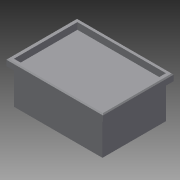
# Autodesk Inventor part: LED_BUTTON
Saved by Autodesk Inventor 2015 (Build 190159000, 159)
## iProperties
Created: 2015-02-07
Part Number: LED_BUTTON
Material: Generic
Document SubType Name: Modeling
Designer: lucanao16
Density: 1 g/cm^3
Appearance: Default
Author: lucanao16
Autodesk Inventor part; units mm, degrees
ref_plane "YZ Plane" through (0, 0, 0) normal (1, 0, 0) x (0, 1, 0)
ref_plane "XZ Plane" through (0, 0, 0) normal (0, 1, 0) x (-1, 0, 0)
ref_plane "XY Plane" through (0, 0, 0) normal (0, 0, 1) x (1, 0, 0)
sketch "Sketch1" plane through (0, 0, 0) normal (0, 1, 0) x (-1, 0, 0)
  line L0 (0, 0) -> (21.9964, 0)
  line L1 (21.9964, 0) -> (21.9964, -15.7734)
  line L2 (21.9964, -15.7734) -> (0, -15.7734)
  line L3 (0, -15.7734) -> (0, 0)
  dimension "d0" = 21.9964
  dimension "d1" = 15.7734
  constraints: 8 end point, 2 parallel, 1 horizontal, 1 perpendicular
  measures "d0" distance of L1.end L2.end
  measures "d1" distance of L0.end L1.end
extrude "Extrusion1" add sketch "Sketch1" along normal blind 8.6868
sketch "Sketch2" plane through (0, 8.6868, 0) normal (0, 1, 0) x (1, 0, 0)
  line L0 (-21.9964, 0) -> (0, 0) projected
  line L1 (0, 0) -> (0, 15.7734) projected
  line L2 (0, 15.7734) -> (-21.9964, 15.7734) projected
  line L3 (-21.9964, 15.7734) -> (-21.9964, 0) projected
  line L4 (-10.9982, 7.8867) -> (-10.9982, 16.6751)
  line L5 (-10.9982, 7.8867) -> (-22.9997, 7.8867)
  line L6 (-22.9997, 16.6751) -> (1.0287, 16.6751)
  line L7 (1.0287, 16.6751) -> (1.0287, -0.9017)
  line L8 (1.0287, -0.9017) -> (-22.9997, -0.9017)
  line L9 (-22.9997, -0.9017) -> (-22.9997, 16.6751)
  dimension "d4" = 8.7884
  dimension "d5" = 12.0015
  dimension "d6" = 24.0284
  dimension "d7" = 17.5768
  dimension "d8" = 0
  dimension "d9" = 7.8867
  constraints: 12 end point, 2 horizontal, 2 parallel, 1 perpendicular, 1 vertical
  measures "d4" distance of L4.start L4.end
  measures "d5" distance of L4.start L5.end
  measures "d6" distance of L7.end L8.end
  measures "d7" distance of L6.end L7.end
  measures "d8" vertical distance of L6.start L4.end
  measures "d9" distance between parallel lines of L5 L2
extrude "Extrusion2" add sketch "Sketch2" along normal blind 1.651 contours L0 L1 L2 L4 L6 L7 L8 L9 L5 L3 | L5 L9 L6 L4 L2 L3
chamfer "Chamfer1" distance 0.254 angle 45 4 edges at (-10.9855, 10.3378, 0.9017) (1.0287, 10.3378, -7.8867) (-10.9855, 10.3378, -16.6751) (-22.9997, 10.3378, -7.8867)
body "Solid1"
